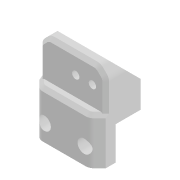
# Autodesk Inventor part: Print_Parts_T
Saved by Autodesk Inventor 2020 (Build 240168000, 168)
## iProperties
Created: 2021-02-11
Part Number: Print_Parts_T
Material: 一般
Document SubType Name: Modeling
Designer: ken113
Density: 1 g/cm^3
Appearance: 既定
Author: ken113
Autodesk Inventor part; units mm, degrees
ref_plane "YZ Plane" through (0, 0, 0) normal (1, 0, 0) x (0, 1, 0)
ref_plane "XZ Plane" through (0, 0, 0) normal (0, 1, 0) x (-1, 0, 0)
ref_plane "XY Plane" through (0, 0, 0) normal (0, 0, 1) x (1, 0, 0)
sketch "スケッチ1" plane through (0, 0, 0) normal (0, 0, 1) x (1, 0, 0)
  line L0 (0, 0) -> (-40, 0)
  line L1 (-40, 0) -> (-40, 51)
  line L2 (-40, 51) -> (0, 51)
  line L3 (0, 51) -> (0, 0)
  dimension "d0" = 51
  dimension "d1" = 40
  constraints: 8 end point, 2 parallel, 1 horizontal, 1 perpendicular
  measures "d0" distance of L0.end L1.end
  measures "d1" distance of L1.end L2.end
extrude "押し出し1" add sketch "スケッチ1" against normal blind 6
sketch "スケッチ2" plane through (0, 0, 0) normal (0, 0, 1) x (1, 0, 0)
  line L0 (0, 51) -> (-40, 51) projected
  point P0 (0, 0)
  point P1 (-8.0667, 39.5)
  point P2 (-18.0667, 39.5)
  dimension "d4" = 10
  dimension "d5" = 11.5
  constraints: 1 horizontal alignment
  measures "d4" distance of point (-8.067, 39.5) point (-18.067, 39.5)
  measures "d5" distance from line of point (-18.067, 39.5) L0
hole "穴1" at (-8.0667, 39.5, 0) at (-18.0667, 39.5, 0) direction (0, 0, -1) diameter 4.4 end through all
sketch "スケッチ3" plane through (0, 0, -6) normal (0, 0, -1) x (-1, 0, 0)
  circle A0 centre (8.0667, 39.5) radius 2.2 projected
  circle A1 centre (18.0667, 39.5) radius 2.2 projected
  line L0 (0, 51) -> (40, 51) projected
  line L1 (40, 51) -> (40, 0) projected
  line L2 (40, 0) -> (0, 0) projected
  line L3 (0, 0) -> (0, 51) projected
  line L4 (0, 0) -> (40, 0) projected
  line L5 (40, 0) -> (40, 51) projected
  line L6 (0, 0) -> (40, 0)
  line L7 (40, 0) -> (40, 20)
  line L8 (40, 20) -> (0, 20)
  line L9 (0, 20) -> (0, 0)
  line L10 (0, 20) -> (40, 20)
  line L11 (40, 20) -> (40, 51)
  line L12 (40, 51) -> (0, 51)
  line L13 (0, 51) -> (0, 20)
  point P0 (0, 20)
  dimension "d13" = 20
  constraints: 16 end point, 4 parallel, 2 horizontal, 2 perpendicular, 1 point on line
  measures "d13" distance between parallel lines of L2 L8
extrude "押し出し2" add sketch "スケッチ3" along normal blind 20 contours A0 | A1 | L0 L1 L8 L3
chamfer "面取り1" distance 20 angle 45 1 edges at (-20, 51, -26)
sketch "スケッチ5" plane through (0, 0, 0) normal (0, 0, 1) x (1, 0, 0)
  circle A0 centre (-8.0667, 39.5) radius 2.2 projected
  circle A1 centre (-18.0667, 39.5) radius 2.2 projected
  line L0 (0, 0) -> (0, 51) projected
  line L1 (0, 51) -> (-40, 51) projected
  line L2 (-40, 51) -> (-40, 0) projected
  line L3 (-40, 0) -> (0, 0) projected
  line L4 (-40, 0) -> (-40, 20) projected
  line L5 (-40, 0) -> (0, 0)
  line L6 (0, 0) -> (0, 28)
  line L7 (0, 28) -> (-40, 28)
  line L8 (-40, 28) -> (-40, 0)
  dimension "d29" = 23
  constraints: 8 end point, 2 parallel, 1 horizontal, 1 perpendicular, 1 point on line
  measures "d29" distance between parallel lines of L1 L7
extrude "押し出し3" add sketch "スケッチ5" along normal blind 5 contours L3 L2 L7 L0
sketch "スケッチ6" plane through (0, 0, 5) normal (0, 0, 1) x (1, 0, 0)
  line L0 (-40, 28) -> (-40, 0) projected
  line L1 (-40, 0) -> (0, 0) projected
  line L2 (0, 0) -> (0, 28) projected
  line L3 (0, 28) -> (-40, 28) projected
  point P0 (-32, 10)
  point P1 (-8, 10)
  dimension "d32" = 10
  dimension "d33" = 8
  dimension "d34" = 8
  constraints: 1 horizontal alignment
  measures "d32" distance from line of point (-32, 10) L1
  measures "d33" distance from line of point (-32, 10) L0
  measures "d34" distance from line of L2 point (-8, 10)
hole "穴3" at (-32, 10, 5) at (-8, 10, 5) direction (0, 0, -1) diameter 4.4 end through all counterbore diameter 8 counterbore depth 7
sketch "スケッチ7" plane through (-40, 51, 0) normal (0, 1, 0) x (1, 0, 0)
  line L0 (0, 6) -> (40, 6) projected
  line L1 (0, 6) -> (0, 26) projected
  line L2 (40, 26) -> (0, 26) projected
  line L3 (40, 6) -> (40, 26) projected
  point P0 (40, 0)
  point P1 (8, 16)
  point P2 (32, 16)
  dimension "d42" = 10
  dimension "d43" = 8
  dimension "d44" = 8
  constraints: 1 horizontal alignment
  measures "d42" distance from line of point (8, 16) L0
  measures "d43" distance from line of L1 point (8, 16)
  measures "d44" distance from line of point (32, 16) L3
hole "穴4" at (-32, 51, -16) at (-8, 51, -16) direction (0, -1, 0) diameter 4.4 end through all counterbore diameter 8 counterbore depth 27
chamfer "面取り2" distance 5 angle 45 6 edges at (0, 14, 5) (-40, 14, 5) (0, 25.5, -26) (-40, 25.5, -26) (0, 51, -3) (-40, 51, -3)
fillet "フィレット1" radius 5 10 edges at (-5, 20.3229, 5) (-5, 3.6771, 5) (-35, 3.6771, 5) (-35, 20.3229, 5) (-40, 46, -5.5) (-35, 51, -3) (-5, 51, -3) (0, 46, -5.5) (-35, 25.5, -26) (-5, 25.5, -26)
chamfer "面取り3" distance 2 angle 45 14 edges at (-20, 28, 5) (-34.8423, 28, 4.6194) (-5.1577, 28, 4.6194) (-38.2322, 28, 1.7678) (-1.7678, 28, 1.7678) (-40, 35.9645, 0) (-39.6194, 45.8423, 0) (-37.5, 48.5, 0) (-2.5, 48.5, 0) (-34.8423, 50.6194, 0) (-5.1577, 50.6194, 0) (-20, 51, 0) (-0.3806, 45.8423, 0) (0, 35.9645, 0)
